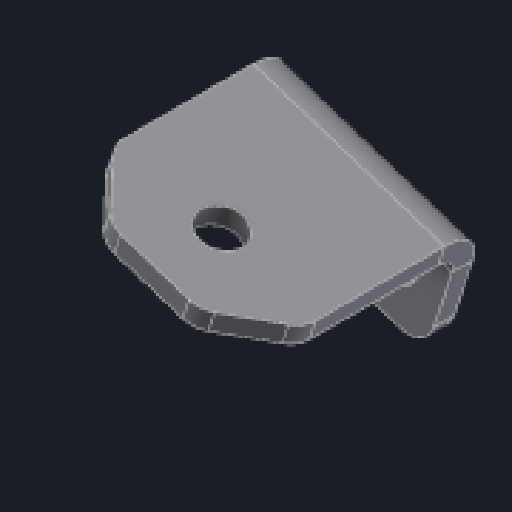
# Autodesk Inventor part: ChestBottomConnector
Saved by Autodesk Inventor 2025.2 (Build 292293000, 293)
## iProperties
Created: 2025-09-26
Part Number: ChestBottomConnector
Material: Generic
Document SubType Name: Sheet Metal
Designer: valer
Density: 1 g/cm^3
Sheet Metal Rule: Default
Appearance: Default
Author: valer
Autodesk Inventor part; units mm, degrees
ref_plane "YZ Plane" through (0, 0, 0) normal (1, 0, 0) x (0, 1, 0)
ref_plane "XZ Plane" through (0, 0, 0) normal (0, 1, 0) x (-1, 0, 0)
ref_plane "XY Plane" through (0, 0, 0) normal (0, 0, 1) x (1, 0, 0)
sketch "Sketch1" plane through (0, 0, 0) normal (0, 0, 1) x (1, 0, 0)
  circle A0 centre (29.4357, 133.8854) radius 3
  circle A1 centre (44.6474, 128.9251) radius 3
  line L0 (-87.8023, 180.5298) -> (92.7626, 121.6499) construction
  line L1 (29.4357, 133.8854) -> (44.6474, 128.9251) construction
  line L2 (25.2608, 143.6614) -> (53.7827, 134.3608)
  line L3 (53.7827, 134.3608) -> (48.8223, 119.1491)
  line L4 (25.2608, 143.6614) -> (20.3004, 128.4497)
  line L5 (20.3004, 128.4497) -> (48.8223, 119.1491)
  line L6 (37.0416, 131.4053) -> (39.5217, 139.0111) construction
  point P0 (0, 0)
  dimension "d0" = 30
  measures "d0" distance of L4.end L3.end
extrude "Plate1" add sketch "Sketch1" along normal blind 3.048
sketch "Sketch2" plane through (26.2057, 146.5592, 0) normal (-0.3100206, -0.9507298, 0) x (0.9507298, -0.3100206, 0)
  line L0 (30, 0) -> (0, 0)
  line L1 (0, 0) -> (0, 35)
  line L2 (0, 35) -> (30, 35)
  line L3 (30, 35) -> (30, 0)
  constraints: 8 end point
edge flange "FlangeFeature" height 35 angle 90 thickness 3.048 bend radius 3.048 thickness toward (-0.3100206, -0.9507298, 0) relief straight relief width 3.048 relief depth 1.524 edges at (39.5217, 139.0111, 3.048) wall of the first edge with corners at (54.7276, 137.2586, 0) (26.2057, 146.5592, 0) (26.2057, 146.5592, 35) (54.7276, 137.2586, 35)
bend "Bend1"
corner "Corner1"
chamfer "ChamferFeature" distance 8 angle 45 2 edges at (25.7332, 145.1103, 35) (54.2551, 135.8097, 35)
fillet "OutsideFilletsFeature" radius 4 6 edges at (25.7332, 145.1103, 27) (33.3391, 142.6301, 35) (46.6493, 138.2899, 35) (54.2551, 135.8097, 27) (20.3004, 128.4497, 1.524) (48.8223, 119.1491, 1.524)
sketch "MountHole" plane through (54.7276, 137.2586, 25.3431) normal (0.3100206, 0.9507298, 0) x (0.9507298, -0.3100206, 0)
  line L0 (0, 19.2471) -> (-30, 19.2471) construction
  line L1 (-15, 19.2471) -> (-15, -9.6569) construction
  line L2 (-9.6569, -9.6569) -> (-20.3431, -9.6569) construction
  circle A0 centre (-15, 0.3431) radius 3.175
  point P0 (-9.4782, 25.3431)
  dimension "d16" = 6.35
  dimension "d17" = 10
  constraints: 2 end point, 2 midpoint, 1 centre point, 1 point on line
  measures "d16" diameter of A0
  measures "d17" distance from line of L2 A0.centre
extrude "MountHoleFeature" cut sketch "MountHole" against normal blind 3.048
equation "\"d18\" = Thickness"
equation "\"d1\" = Thickness"
equation "\"d2\" = BendReliefWidth"
equation "\"d3\" = BendReliefDepth"
equation "\"d4\" = MinimumRemnant"
equation "\"d5\" = TransitionRadius"
equation "\"d8\" = BendRadius"
equation "\"d9\" = CornerReliefSize"
equation "\"d10\" = GapSize"
equation "\"d11\" = JacobiRadiusSize"
equation "\"BendRadius\" = Thickness"
equation "\"BendReliefWidth\" = Thickness"
equation "\"BendReliefDepth\" = 0.5 * Thickness"
equation "\"CornerReliefSize\" = 4 * Thickness"
equation "\"MinimumRemnant\" = 2 * Thickness"
equation "\"TransitionRadius\" = BendRadius"
equation "\"JacobiRadiusSize\" = BendRadius"
equation "\"GapSize\" = Thickness"
equation "\"Thickness\" = 3.048"
body "Solid1"
